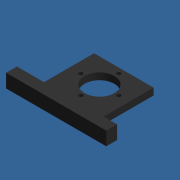
# Autodesk Inventor part: Shoulder_stepper_holder
Saved by Autodesk Inventor 2016 (Build 200138000, 138)
## iProperties
Created: 2015-02-18
Part Number: Shoulder_stepper_holder
Material: ABS-Kunststoff - Schwarz
Document SubType Name: Modeling
Designer: 4ndreas
Density: 1.06 g/cm^3
Appearance: Glatt - weiß(2)
Author: 4ndreas
Autodesk Inventor part; units mm, degrees
ref_plane "YZ Plane" through (0, 0, 0) normal (1, 0, 0) x (0, 1, 0)
ref_plane "XZ Plane" through (0, 0, 0) normal (0, 1, 0) x (-1, 0, 0)
ref_plane "XY Plane" through (0, 0, 0) normal (0, 0, 1) x (1, 0, 0)
sketch "Skizze1" plane through (0, 0, 0) normal (0, 0, 1) x (1, 0, 0)
  line L0 (-0.2717, 2) -> (-0.2717, -2.4631) projected
  arc A0 (-2.2717, 0) -> (-0.2717, 2) centre (-2.2717, 2) ccw projected
  line L1 (-42.2717, 0) -> (-2.2717, 0) projected
  arc A1 (-44.2717, 2) -> (-42.2717, 0) centre (-42.2717, 2) ccw projected
  line L2 (-44.2717, 2) -> (-44.2717, -2.4631) projected
  line L3 (-44.2717, -2.4631) -> (-59.2717, -2.4631) projected
  line L4 (-59.2717, -10.4631) -> (-59.2717, -2.4631) projected
  line L5 (-37.1489, -10.4631) -> (-59.2717, -10.4631) projected
  line L6 (-37.1489, -7.4631) -> (-37.1489, -10.4631) projected
  line L7 (-26.4444, -7.4631) -> (-37.1489, -7.4631) projected
  line L8 (-26.4444, -10.4631) -> (-26.4444, -7.4631) projected
  line L9 (-18.0989, -10.4631) -> (-26.4444, -10.4631) projected
  line L10 (-18.0989, -7.4631) -> (-18.0989, -10.4631) projected
  line L11 (-7.3944, -7.4631) -> (-18.0989, -7.4631) projected
  line L12 (-7.3944, -10.4631) -> (-7.3944, -7.4631) projected
  line L13 (14.7283, -10.4631) -> (-7.3944, -10.4631) projected
  line L14 (14.7283, -10.4631) -> (14.7283, -2.4631) projected
  line L15 (14.7283, -2.4631) -> (-0.2717, -2.4631) projected
  circle A2 centre (-22, 7.4835) radius 1.5 projected
  circle A3 centre (-36, 21.4835) radius 1.5 projected
  circle A4 centre (-22, 35.4835) radius 1.5 projected
  circle A5 centre (-8, 21.4835) radius 1.5 projected
  circle A6 centre (-22, 21.4835) radius 18 projected
  circle A7 centre (-22, 21.4835) radius 11 projected
  line L16 (-44.2717, -10.4631) -> (-0.2717, -10.4631)
  line L17 (-0.2717, -10.4631) -> (-0.2717, 39.4835)
  line L18 (-0.2717, 39.4835) -> (-44.2717, 39.4835)
  line L19 (-44.2717, 39.4835) -> (-44.2717, -10.4631)
  point P0 (0, 0)
  constraints: 8 end point, 3 collinear, 2 parallel, 1 horizontal, 1 perpendicular, 1 tangent
extrude "Extrusion1" add sketch "Skizze1" along normal blind 5 contours L0 L17 L13 L12 L11 L10 L9 L8 L7 L6 L5 L19 L2 A1 L1 A0 | A6 | A0 L1 A1 L19 L18 L17 | L15 L14 L13 L17 | L16 L10 L11 L12 | L19 L5 L4 L3 | L16 L6 L7 L8
sketch "Skizze2" plane through (0, 0, 5) normal (0, 0, 1) x (1, 0, 0)
  line L0 (-59.2717, -10.4631) -> (14.7283, -10.4631) projected
  line L1 (14.7283, -10.4631) -> (14.7283, -2.4631) projected
  line L2 (-59.2717, -10.4631) -> (14.7283, -10.4631)
  line L3 (14.7283, -10.4631) -> (14.7283, -2.4631)
  line L4 (14.7283, -2.4631) -> (-59.2717, -2.4631)
  line L5 (-59.2717, -2.4631) -> (-59.2717, -10.4631)
  point P0 (0, 0)
  constraints: 8 end point, 2 parallel, 1 horizontal, 1 perpendicular
extrude "Extrusion2" add sketch "Skizze2" along normal blind 5
